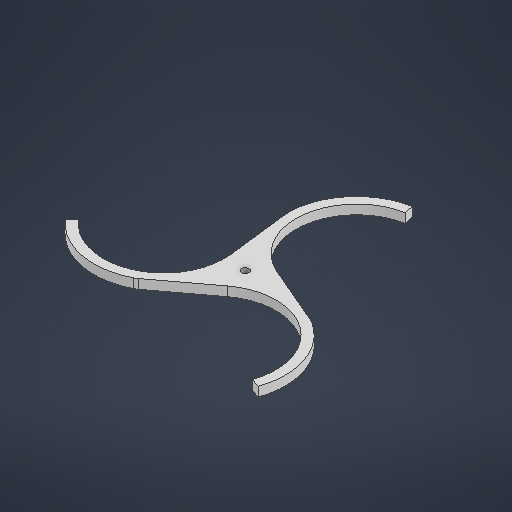
# Autodesk Inventor part: сюрикен
Saved by Autodesk Inventor 2026.2 (Build 302298000, 298)
## iProperties
Created: 2025-11-21
Part Number: сюрикен
Material: Типовые
Document SubType Name: Modeling
Designer: Phantom
Density: 1 g/cm^3
Appearance: По умолчанию
Author: Phantom
Autodesk Inventor part; units mm, degrees
ref_plane "YZ Plane" through (0, 0, 0) normal (1, 0, 0) x (0, 1, 0)
ref_plane "XZ Plane" through (0, 0, 0) normal (0, 1, 0) x (-1, 0, 0)
ref_plane "XY Plane" through (0, 0, 0) normal (0, 0, 1) x (1, 0, 0)
sketch "Эскиз1" plane through (0, 0, 0) normal (0, 1, 0) x (-1, 0, 0)
  circle A0 centre (0, 0) radius 152.5
  line L0 (0, 0) -> (152.5, 0)
  circle A1 centre (87.5, 0) radius 65
  circle A2 centre (-43.75, 75.777223) radius 65
  circle A3 centre (-43.75, -75.777223) radius 65
  circle A4 centre (87.5, 0) radius 75
  circle A5 centre (-43.75, 75.777223) radius 75
  circle A6 centre (-43.75, -75.777223) radius 75
  line L1 (0, 0) -> (-76.25, 132.068874)
  line L2 (0, 0) -> (-76.25, -132.068874)
  line L3 (144.5, 48.74423) -> (30.5, -48.74423)
  line L4 (-114.463742, 100.768556) -> (26.963742, 50.78589)
  line L5 (-30.036258, -149.512786) -> (-57.463742, -2.04166)
  line L6 (30.5, -48.74423) -> (26.963742, -50.78589)
  line L7 (26.963742, 50.78589) -> (30.5, 48.74423)
  line L8 (-57.463742, -2.04166) -> (-57.463742, 2.04166)
  point P0 (14.069297, 24.368737)
  point P1 (-28.138593, 0)
  point P2 (14.069297, -24.368737)
  point P3 (12.5, 0)
  point P4 (22.5, 0)
  point P5 (152.5, 0)
  point P6 (-6.25, 10.825318)
  point P7 (-11.25, 19.485572)
  point P8 (-76.25, 132.068874)
  point P9 (-114.463742, 100.768556)
  point P10 (-6.25, -10.825318)
  point P11 (-11.25, -19.485572)
  point P12 (-76.25, -132.068874)
  point P13 (-30.036258, -149.512786)
  point P14 (-114.463742, -100.768556)
  point P15 (-30.036258, 149.512786)
  point P16 (144.5, -48.74423)
  point P17 (152.5, 0)
  point P18 (136.9, 42.245)
  point P19 (17.535243, 54.118068)
  point P20 (-105.035243, 97.436378)
  point P21 (-114.463742, 100.768556)
  point P22 (-57.463742, -2.04166)
  point P23 (-55.635243, -11.873068)
  point P24 (-31.864757, -139.681378)
  point P25 (-30.036258, -149.512786)
  point P26 (38.1, -42.245)
  dimension "d0" = 305
  dimension "d1" = 130
  dimension "d2" = 0
  dimension "d5" = 360
  dimension "d7" = 150
  dimension "d10" = 360
  dimension "d16" = 360
  dimension "d18" = 0
  dimension "d21" = 360
  dimension "d25" = 360
  constraints: 18 end point, 6 centre point, 4 coincident, 4 point on circle, 1 horizontal, 1 tangent, 48 other
  measures "d0" diameter of A0
  measures "d1" diameter of A1
  measures "d2" distance from line of L0 A1.centre
  measures "d7" diameter of A4
  measures "d18" distance from line of A1.centre L3
sketch "Эскиз1 outline for Выдавливание1" plane through (0, 0, 0) normal (0, 1, 0) x (-1, 0, 0)
  line L0 (136.9, 42.245) -> (144.5, 48.74423)
  arc A0 (38.1, -42.245) -> (136.9, 42.245) centre (87.5, 0) cw
  line L1 (30.5, -48.74423) -> (38.1, -42.245)
  line L2 (26.963742, -50.78589) -> (30.5, -48.74423)
  arc A1 (-30.036258, -149.512786) -> (26.963742, -50.78589) centre (-43.75, -75.777223) ccw
  line L3 (-31.864757, -139.681378) -> (-30.036258, -149.512786)
  arc A2 (-55.635243, -11.873068) -> (-31.864757, -139.681378) centre (-43.75, -75.777223) cw
  line L4 (-57.463742, -2.04166) -> (-55.635243, -11.873068)
  line L5 (-57.463742, 2.04166) -> (-57.463742, -2.04166)
  arc A3 (-114.463742, 100.768556) -> (-57.463742, 2.04166) centre (-43.75, 75.777223) ccw
  line L6 (-105.035243, 97.436378) -> (-114.463742, 100.768556)
  arc A4 (17.535243, 54.118068) -> (-105.035243, 97.436378) centre (-43.75, 75.777223) cw
  line L7 (26.963742, 50.78589) -> (17.535243, 54.118068)
  line L8 (30.5, 48.74423) -> (26.963742, 50.78589)
  arc A5 (144.5, 48.74423) -> (30.5, 48.74423) centre (87.5, 0) ccw
extrude "Выдавливание1" add sketch "Эскиз1 outline for Выдавливание1" along normal blind 10
chamfer "Фаска1" distance 10 angle 45 3 edges at (55.6352, 5, -11.8731) (-17.5352, 5, 54.1181) (-38.1, 5, -42.245)
sketch "Эскиз2" plane through (0, 10, 0) normal (0, 1, 0) x (1, 0, 0)
  line L0 (-32.204642, 34.167577) -> (-30.5, 48.74423)
  line L1 (-32.204642, 34.167577) -> (-31.020127, 86.842802)
  arc A0 (30.036258, 149.512786) -> (-26.963742, 50.78589) centre (43.75, 75.777223) ccw
  line L2 (-13.487669, -44.973827) -> (-59.698009, -70.285619)
  line L3 (45.692311, 10.806249) -> (90.718136, -16.557183)
  line L4 (-32.204642, 34.167577) -> (-30.5, 48.74423)
  arc A1 (-136.9, -42.245) -> (-32.204642, 34.167577) centre (-87.5, 0) ccw
  line L5 (-136.9, -42.245) -> (-144.5, -48.74423)
  arc A2 (-144.5, -48.74423) -> (-30.5, -48.74423) centre (-87.5, 0) ccw
  line L6 (-30.5, -48.74423) -> (-26.963742, -50.78589)
  line L7 (-13.487669, -44.973827) -> (-26.963742, -50.78589)
  arc A3 (105.035243, -97.436378) -> (-13.487669, -44.973827) centre (43.75, -75.777223) ccw
  line L8 (105.035243, -97.436378) -> (114.463742, -100.768556)
  arc A4 (114.463742, -100.768556) -> (57.463742, -2.04166) centre (43.75, -75.777223) ccw
  line L9 (57.463742, -2.04166) -> (57.463742, 2.04166)
  line L10 (45.692311, 10.806249) -> (57.463742, 2.04166)
  arc A5 (31.864757, 139.681378) -> (45.692311, 10.806249) centre (43.75, 75.777223) ccw
  line L11 (31.864757, 139.681378) -> (30.036258, 149.512786)
  arc A6 (30.036258, 149.512786) -> (-26.963742, 50.78589) centre (43.75, 75.777223) ccw
  line L12 (-26.963742, 50.78589) -> (-30.5, 48.74423)
  point P0 (0, 0)
  point P1 (82.700735, -11.684788)
  point P2 (-51.46969, -65.778544)
  point P3 (-31.231045, 77.463331)
  dimension "d32" = 360
  constraints: 6 end point, 1 tangent, 10 other
sketch "Эскиз2 outline for Выдавливание2" plane through (0, 10, 0) normal (0, 1, 0) x (1, 0, 0)
  line L0 (57.463742, 2.04166) -> (57.463742, -2.04166)
  line L1 (45.692311, 10.806249) -> (57.463742, 2.04166)
  line L2 (82.700735, -11.684788) -> (45.692311, 10.806249)
  arc A0 (57.463742, -2.04166) -> (82.700735, -11.684788) centre (43.75, -75.777223) cw
  line L3 (-26.963742, -50.78589) -> (-30.5, -48.74423)
  line L4 (-13.487669, -44.973827) -> (-26.963742, -50.78589)
  line L5 (-51.46969, -65.778544) -> (-13.487669, -44.973827)
  arc A1 (-30.5, -48.74423) -> (-51.46969, -65.778544) centre (-87.5, 0) cw
  line L6 (-30.5, 48.74423) -> (-26.963742, 50.78589)
  line L7 (-32.204642, 34.167577) -> (-30.5, 48.74423)
  line L8 (-31.231045, 77.463331) -> (-32.204642, 34.167577)
  arc A2 (-26.963742, 50.78589) -> (-31.231045, 77.463331) centre (43.75, 75.777223) cw
extrude "Выдавливание2" add sketch "Эскиз2 outline for Выдавливание2" against normal blind 10
sketch "Эскиз3" plane through (0, 10, 0) normal (0, 1, 0) x (1, 0, 0)
  arc A0 (-136.9, -42.245) -> (-32.204642, 34.167577) centre (-87.5, 0) ccw
  line L0 (-136.9, -42.245) -> (-144.5, -48.74423)
  arc A1 (-144.5, -48.74423) -> (-51.46969, -65.778544) centre (-87.5, 0) ccw
  line L1 (-51.46969, -65.778544) -> (-13.487669, -44.973827)
  arc A2 (105.035243, -97.436378) -> (-13.487669, -44.973827) centre (43.75, -75.777223) ccw
  line L2 (105.035243, -97.436378) -> (114.463742, -100.768556)
  arc A3 (114.463742, -100.768556) -> (82.700735, -11.684788) centre (43.75, -75.777223) ccw
  line L3 (82.700735, -11.684788) -> (45.692311, 10.806249)
  arc A4 (31.864757, 139.681378) -> (45.692311, 10.806249) centre (43.75, 75.777223) ccw
  line L4 (31.864757, 139.681378) -> (30.036258, 149.512786)
  arc A5 (30.036258, 149.512786) -> (-31.231045, 77.463331) centre (43.75, 75.777223) ccw
  line L5 (-31.231045, 77.463331) -> (-32.204642, 34.167577)
  line L6 (-31.231045, 77.463331) -> (-15.37541, -56.235706)
  line L7 (-51.46969, -65.778544) -> (56.389255, 14.802358)
  line L8 (82.700735, -11.684788) -> (-41.013845, 41.433348)
  point P0 (0, 0)
  point P1 (4.846874, -23.704708)
  point P2 (18.105443, 16.04987)
  point P3 (-22.952316, 7.654838)
  dimension "d38" = 360
  constraints: 6 end point, 1 tangent, 10 other
sketch "Эскиз3 outline for Выдавливание3" plane through (0, 10, 0) normal (0, 1, 0) x (1, 0, 0)
  line L0 (4.846874, -23.704708) -> (-51.46969, -65.778544)
  arc A0 (-13.487669, -44.973827) -> (4.846874, -23.704708) centre (43.75, -75.777223) cw
  line L1 (-51.46969, -65.778544) -> (-13.487669, -44.973827)
  line L2 (18.105443, 16.04987) -> (82.700735, -11.684788)
  arc A1 (45.692311, 10.806249) -> (18.105443, 16.04987) centre (43.75, 75.777223) cw
  line L3 (82.700735, -11.684788) -> (45.692311, 10.806249)
  line L4 (-22.952316, 7.654838) -> (-31.231045, 77.463331)
  arc A2 (-32.204642, 34.167577) -> (-22.952316, 7.654838) centre (-87.5, 0) cw
  line L5 (-31.231045, 77.463331) -> (-32.204642, 34.167577)
extrude "Выдавливание3" cut sketch "Эскиз3 outline for Выдавливание3" against normal through all
fillet "Сопряжение1" radius 20 3 edges at (82.7007, 5, 11.6848) (-51.4697, 5, 65.7785) (-31.231, 5, -77.4633)
sketch "Эскиз4" plane through (0, 10, 0) normal (0, 1, 0) x (1, 0, 0)
  circle A0 centre (0, 0) radius 4
  dimension "d43" = 8
  constraints: 1 centre point, 1 coincident
  measures "d43" diameter of A0
sketch "Эскиз4 outline for Выдавливание4" plane through (0, 10, 0) normal (0, 1, 0) x (1, 0, 0)
  circle A0 centre (0, 0) radius 4
extrude "Выдавливание4" cut sketch "Эскиз4 outline for Выдавливание4" against normal blind 140
